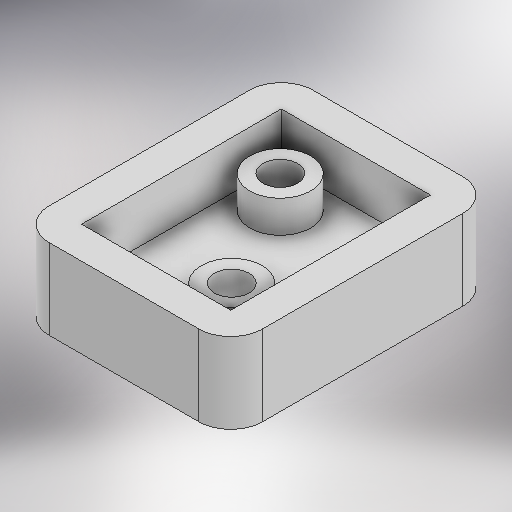
# Autodesk Inventor part: environmental_sensor_case
Saved by Autodesk Inventor 2026 (Build 300175050, 175E)
## iProperties
Created: 2025-09-30
Part Number: environmental_sensor_case
Material: Generic
Document SubType Name: Modeling
Designer: satom
Density: 1 g/cm^3
Appearance: Default
Author: satom
Autodesk Inventor part; units mm, degrees
ref_plane "YZ Plane" through (0, 0, 0) normal (1, 0, 0) x (0, 1, 0)
ref_plane "XZ Plane" through (0, 0, 0) normal (0, 1, 0) x (-1, 0, 0)
ref_plane "XY Plane" through (0, 0, 0) normal (0, 0, 1) x (1, 0, 0)
sketch "Sketch1" plane through (0, 0, 0) normal (0, 1, 0) x (-1, 0, 0)
  line L0 (-10.55, -13.05) -> (10.55, -13.05)
  line L1 (10.55, -13.05) -> (10.55, 13.05)
  line L2 (10.55, 13.05) -> (-10.55, 13.05)
  line L3 (-10.55, 13.05) -> (-10.55, -13.05)
  line L4 (-10.55, -13.05) -> (10.55, 13.05) construction
  line L5 (10.55, -13.05) -> (-10.55, 13.05) construction
  point P0 (0, 0)
  dimension "d0" = 26.1
  dimension "d1" = 21.1
  constraints: 12 end point, 2 midpoint, 2 parallel, 1 horizontal, 1 perpendicular
  measures "d0" distance of L0.end L1.end
  measures "d1" distance of L1.end L2.end
extrude "Extrusion1" add sketch "Sketch1" along normal blind 7.95
sketch "Sketch2" plane through (0, 7.95, 0) normal (0, 1, 0) x (1, 0, 0)
  line L0 (7.375, -9.875) -> (-7.375, -9.875)
  line L1 (-7.375, -9.875) -> (-7.375, 9.875)
  line L2 (-7.375, 9.875) -> (7.375, 9.875)
  line L3 (7.375, 9.875) -> (7.375, -9.875)
  line L4 (7.375, -9.875) -> (-7.375, 9.875) construction
  line L5 (-7.375, -9.875) -> (7.375, 9.875) construction
  point P0 (0, 0)
  dimension "d4" = 19.75
  dimension "d5" = 14.75
  constraints: 12 end point, 2 midpoint, 2 parallel, 1 horizontal, 1 perpendicular
  measures "d4" distance of L0.end L1.end
  measures "d5" distance of L0.start L0.end
extrude "Extrusion2" cut sketch "Sketch2" against normal blind 4.775
sketch "Sketch3" plane through (0, 3.175, 0) normal (0, 1, 0) x (1, 0, 0)
  circle A0 centre (-3.5, 5.9) radius 3
  circle A1 centre (3.5, -5.9) radius 3
  point P0 (0, 0)
  dimension "d8" = 11.8
  dimension "d9" = 7
  dimension "d10" = 5.9
  dimension "d11" = 3.5
  dimension "d12" = 6
  dimension "d13" = 6
  constraints: 2 centre point
  measures "d8" vertical distance of A1.centre A0.centre
  measures "d9" horizontal distance of A1.centre A0.centre
  measures "d10" vertical distance of point (0, 0) A0.centre
  measures "d11" horizontal distance of point (0, 0) A0.centre
  measures "d12" diameter of A0
  measures "d13" diameter of A1
extrude "Extrusion3" add sketch "Sketch3" along normal blind 3.175
sketch "Sketch4" plane through (3.5, 6.35, 5.9) normal (0, 1, 0) x (1, 0, 0)
  circle A0 centre (0, 0) radius 1.7
  circle A1 centre (-7, 11.8) radius 3 projected
  circle A2 centre (-7, 11.8) radius 1.7
  point P0 (-3.5, 5.9)
  dimension "d16" = 3.4
  dimension "d17" = 3.4
  constraints: 2 centre point, 1 coincident
  measures "d16" diameter of A0
  measures "d17" diameter of A2
extrude "Extrusion4" cut sketch "Sketch4" against normal through all contours A0 | A2
fillet "Fillet1" radius 3.175 4 edges at (10.55, 3.975, 13.05) (10.55, 3.975, -13.05) (-10.55, 3.975, 13.05) (-10.55, 3.975, -13.05)
equation "\"d10\" = 0.5 * d8"
equation "\"d11\" = 0.5 * d9"
equation "\"d13\" = d12"
equation "\"d16\" = m3_clearance"
equation "\"d17\" = m3_clearance"
equation "\"m3_heat_set_insert\" = 4"
equation "\"m3_clearance\" = 3.4"
equation "\"m3_heat_set_depth\" = 7"
equation "\"robot_diameter\" = 354"
equation "\"hardboard_thickness\" = 5"
equation "\"motor_centerline_height\" = 13"
body "Solid1"
